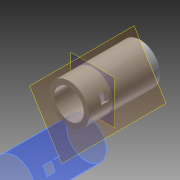
# Autodesk Inventor part: PVC Spacer 500 Sched 40
Saved by Autodesk Inventor 2013 (Build 170138000, 138)
## iProperties
Created: 2013-04-06
Part Number: PVC Spacer 500 Sched 40
Material: PVC-Piping
Document SubType Name: Modeling
Designer: Niemitalo_Dan
Density: 1 g/cm^3
Author: Niemitalo_Dan
Autodesk Inventor part; units mm, degrees
ref_plane "YZ Plane" through (0, 0, 0) normal (1, 0, 0) x (0, 1, 0)
ref_plane "XZ Plane" through (0, 0, 0) normal (0, 1, 0) x (-1, 0, 0)
ref_plane "XY Plane" through (0, 0, 0) normal (0, 0, 1) x (1, 0, 0)
sketch "Sketch1" plane through (0, 0, 0) normal (0, 0, 1) x (1, 0, 0)
  circle A0 centre (0, 0) radius 7.8994
  circle A1 centre (0, 0) radius 10.668
  dimension "d0" = 15.7988
  dimension "d2" = 21.336
  constraints: 2 centre point, 2 coincident
  measures "d0" diameter of A0
  measures "d2" diameter of A1
extrude "Extrusion1" add sketch "Sketch1" along normal mid plane 38.1
ref_plane "Work Plane1" through (0, 0, 6.35) normal (0, 0, -1) x (-1, 0, 0)
sketch "Sketch3" plane through (0, 0, 6.35) normal (0, 0, -1) x (-1, 0, 0)
  line L0 (-7.3505, 7.6359) -> (-5.5315, 5.6464)
  line L1 (-5.5315, 5.6464) -> (-7.3505, 7.6359)
  line L2 (-6.8389, 3.8843) -> (-9.0558, 5.6464)
  arc A0 (-7.3505, 7.6359) -> (-9.0558, 5.6464) centre (5.6213, -5.2084) ccw
  arc A1 (-5.5315, 5.6464) -> (-6.8389, 3.8843) centre (-5.2401, 4.0642) ccw
  point P0 (0, 0)
  constraints: 6 end point, 4 point on circle, 2 centre point, 1 collinear
extrude "Extrusion3" cut sketch "Sketch3" along normal blind 3.175
ref_plane "Work Plane3" through (9.0527, 5.644, 0) normal (0.8485864, 0.5290569, 0) x (-0.5290569, 0.8485864, 0)
sketch "Sketch4" plane through (9.0527, 5.644, 0) normal (0.8485864, 0.5290569, 0) x (-0.5290569, 0.8485864, 0)
  line L0 (0, 12.2855) -> (0, 7.9748)
  line L1 (0, 7.9748) -> (-4.4544, 7.9748)
  line L2 (-4.4544, 7.9748) -> (-4.4544, 12.2855)
  line L3 (-4.4544, 12.2855) -> (0, 12.2855)
  point P0 (0, 0)
  constraints: 8 end point, 2 parallel, 1 perpendicular, 1 vertical
extrude "Extrusion4" cut sketch "Sketch4" against normal blind 6.35
body "Solid1"
